Autodesk Fusion 360 part; units mm, degrees
(part 3 of 6)
  line L1098 (9.2939, 42.25) -> (5.0046, 42.25)
  line L1099 (4.1969, 48.5626) -> (3.4334, 47.8252)
  line L1100 (5.015, 40.75) -> (3.5, 40.75)
  line L1101 (3.5, 40.75) -> (2.5142, 47.7125)
  line L1102 (8.8126, 47.0763) -> (9.7083, 40.75)
  line L1103 (9.5063, 40.75) -> (9.2939, 42.25)
  line L1104 (8.5104, 47.0626) -> (9.274, 47.7999)
  line L1105 (10.1943, 47.9115) -> (9.4443, 47.9115)
  line L1106 (11.2083, 40.75) -> (10.2224, 47.7135)
  arc A162 (2.0758, 54.875) -> (1.5807, 54.3049) centre (2.0758, 54.375) ccw
  line L1107 (5.217, 40.75) -> (9.5063, 40.75)
  line L1108 (4.1602, 46.7869) -> (5.015, 40.75)
  line L1109 (9.4724, 47.7135) -> (8.8126, 47.0763)
  line L1110 (5.0046, 42.25) -> (5.217, 40.75)
  line L1111 (4.1717, 47.0626) -> (8.5104, 47.0626)
  line L1112 (9.4443, 47.9115) -> (8.5483, 48.8371)
  line L1113 (2.5142, 47.7125) -> (3.2642, 47.7125)
  line L1114 (10.2224, 47.7135) -> (9.4724, 47.7135)
  arc A163 (3.4391, 41.1799) -> (3.9342, 40.75) centre (3.9342, 41.25) ccw
  line L1115 (3.2358, 47.9125) -> (2.4858, 47.9125)
  line L1116 (7.4934, 54.875) -> (7.7058, 53.375)
  arc A164 (9.2692, 54.4451) -> (8.7741, 54.875) centre (8.7741, 54.375) ccw
  line L1117 (2.4858, 47.9125) -> (1.5, 54.875)
  line L1118 (3.4274, 53.375) -> (3.215, 54.875)
  line L1119 (9.2083, 54.875) -> (10.1943, 47.9115)
  line L1120 (3.4334, 47.8252) -> (4.1717, 47.0626)
  line L1121 (3.015, 54.875) -> (3.9088, 48.5624)
  line L1122 (9.274, 47.7999) -> (8.5357, 48.5626)
  line L1123 (8.5483, 48.8371) -> (7.6934, 54.875)
  line L1124 (3.215, 54.875) -> (7.4934, 54.875)
  line L1125 (8.5357, 48.5626) -> (4.1969, 48.5626)
  line L1126 (7.6934, 54.875) -> (9.2083, 54.875)
  line L1127 (3.9088, 48.5624) -> (3.2358, 47.9125)
  line L1128 (20.4138, 53.375) -> (16.1354, 53.375)
  line L1129 (15.723, 54.875) -> (14.208, 54.875)
  arc A165 (23.3405, 40.75) -> (23.8356, 41.3201) centre (23.3405, 41.25) ccw
  circle A166 centre (14.208, 41.625) radius 0.875
  line L1130 (15.9722, 47.7125) -> (16.8682, 46.7869)
  line L1131 (22.4163, 40.75) -> (23.9163, 40.75)
  line L1132 (22.0019, 42.25) -> (17.7126, 42.25)
  line L1133 (16.9049, 48.5626) -> (16.1414, 47.8252)
  line L1134 (17.723, 40.75) -> (16.208, 40.75)
  line L1135 (16.208, 40.75) -> (15.2222, 47.7125)
  line L1136 (21.5206, 47.0763) -> (22.4163, 40.75)
  line L1137 (22.2143, 40.75) -> (22.0019, 42.25)
  line L1138 (21.2184, 47.0626) -> (21.982, 47.7999)
  line L1139 (22.9023, 47.9115) -> (22.1523, 47.9115)
  line L1140 (23.9163, 40.75) -> (22.9304, 47.7135)
  arc A167 (14.7838, 54.875) -> (14.2887, 54.3049) centre (14.7838, 54.375) ccw
  line L1141 (17.925, 40.75) -> (22.2143, 40.75)
  line L1142 (16.8682, 46.7869) -> (17.723, 40.75)
  line L1143 (22.1804, 47.7135) -> (21.5206, 47.0763)
  line L1144 (17.7126, 42.25) -> (17.925, 40.75)
  line L1145 (16.8797, 47.0626) -> (21.2184, 47.0626)
  line L1146 (22.1523, 47.9115) -> (21.2563, 48.8371)
  line L1147 (15.2222, 47.7125) -> (15.9722, 47.7125)
  line L1148 (22.9304, 47.7135) -> (22.1804, 47.7135)
  arc A168 (16.1471, 41.1799) -> (16.6422, 40.75) centre (16.6422, 41.25) ccw
  line L1149 (15.9438, 47.9125) -> (15.1938, 47.9125)
  line L1150 (20.2014, 54.875) -> (20.4138, 53.375)
  arc A169 (21.9772, 54.4451) -> (21.4821, 54.875) centre (21.4821, 54.375) ccw
  line L1151 (15.1938, 47.9125) -> (14.208, 54.875)
  line L1152 (16.1354, 53.375) -> (15.923, 54.875)
  line L1153 (21.9163, 54.875) -> (22.9023, 47.9115)
  line L1154 (16.1414, 47.8252) -> (16.8797, 47.0626)
  line L1155 (15.723, 54.875) -> (16.6168, 48.5624)
  line L1156 (21.982, 47.7999) -> (21.2437, 48.5626)
  line L1157 (21.2563, 48.8371) -> (20.4014, 54.875)
  line L1158 (15.923, 54.875) -> (20.2014, 54.875)
  line L1159 (21.2437, 48.5626) -> (16.9049, 48.5626)
  line L1160 (20.4014, 54.875) -> (21.9163, 54.875)
  line L1161 (16.6168, 48.5624) -> (15.9438, 47.9125)
  line L1162 (33.1218, 53.375) -> (28.8434, 53.375)
  line L1163 (28.431, 54.875) -> (26.916, 54.875)
  arc A170 (36.0485, 40.75) -> (36.5436, 41.3201) centre (36.0485, 41.25) ccw
  circle A171 centre (26.916, 41.625) radius 0.875
  line L1164 (28.6802, 47.7125) -> (29.5762, 46.7869)
  line L1165 (35.1243, 40.75) -> (36.6243, 40.75)
  line L1166 (34.7099, 42.25) -> (30.4206, 42.25)
  line L1167 (29.6129, 48.5626) -> (28.8494, 47.8252)
  line L1168 (30.431, 40.75) -> (28.916, 40.75)
  line L1169 (28.916, 40.75) -> (27.9302, 47.7125)
  line L1170 (34.2286, 47.0763) -> (35.1243, 40.75)
  line L1171 (34.9223, 40.75) -> (34.7099, 42.25)
  line L1172 (33.9264, 47.0626) -> (34.69, 47.7999)
  line L1173 (35.6103, 47.9115) -> (34.8603, 47.9115)
  line L1174 (36.6243, 40.75) -> (35.6384, 47.7135)
  arc A172 (27.4918, 54.875) -> (26.9967, 54.3049) centre (27.4918, 54.375) ccw
  line L1175 (30.633, 40.75) -> (34.9223, 40.75)
  line L1176 (29.5762, 46.7869) -> (30.431, 40.75)
  line L1177 (34.8884, 47.7135) -> (34.2286, 47.0763)
  line L1178 (30.4206, 42.25) -> (30.633, 40.75)
  line L1179 (29.5877, 47.0626) -> (33.9264, 47.0626)
  line L1180 (34.8603, 47.9115) -> (33.9643, 48.8371)
  line L1181 (27.9302, 47.7125) -> (28.6802, 47.7125)
  line L1182 (35.6384, 47.7135) -> (34.8884, 47.7135)
  arc A173 (28.8551, 41.1799) -> (29.3502, 40.75) centre (29.3502, 41.25) ccw
  line L1183 (28.6518, 47.9125) -> (27.9018, 47.9125)
  line L1184 (32.9094, 54.875) -> (33.1218, 53.375)
  arc A174 (34.6852, 54.4451) -> (34.1901, 54.875) centre (34.1901, 54.375) ccw
  line L1185 (27.9018, 47.9125) -> (26.916, 54.875)
  line L1186 (28.8434, 53.375) -> (28.631, 54.875)
  line L1187 (34.6243, 54.875) -> (35.6103, 47.9115)
  line L1188 (28.8494, 47.8252) -> (29.5877, 47.0626)
  line L1189 (28.431, 54.875) -> (29.3248, 48.5624)
  line L1190 (34.69, 47.7999) -> (33.9517, 48.5626)
  line L1191 (33.9643, 48.8371) -> (33.1094, 54.875)
  line L1192 (28.631, 54.875) -> (32.9094, 54.875)
  line L1193 (33.9517, 48.5626) -> (29.6129, 48.5626)
  line L1194 (33.1094, 54.875) -> (34.6243, 54.875)
  line L1195 (29.3248, 48.5624) -> (28.6518, 47.9125)
  line L1196 (45.8298, 53.375) -> (41.5514, 53.375)
  line L1197 (41.139, 54.875) -> (39.624, 54.875)
  arc A175 (48.7565, 40.75) -> (49.2516, 41.3201) centre (48.7565, 41.25) ccw
  circle A176 centre (39.624, 41.625) radius 0.875
  line L1198 (41.3882, 47.7125) -> (42.2842, 46.7869)
  line L1199 (47.8323, 40.75) -> (49.3323, 40.75)
  line L1200 (47.4179, 42.25) -> (43.1286, 42.25)
  line L1201 (42.3209, 48.5626) -> (41.5574, 47.8252)
  line L1202 (43.139, 40.75) -> (41.624, 40.75)
  line L1203 (41.624, 40.75) -> (40.6382, 47.7125)
  line L1204 (46.9366, 47.0763) -> (47.8323, 40.75)
  line L1205 (47.6303, 40.75) -> (47.4179, 42.25)
  line L1206 (46.6344, 47.0626) -> (47.398, 47.7999)
  line L1207 (48.3183, 47.9115) -> (47.5683, 47.9115)
  line L1208 (49.3323, 40.75) -> (48.3464, 47.7135)
  arc A177 (40.1998, 54.875) -> (39.7047, 54.3049) centre (40.1998, 54.375) ccw
  line L1209 (43.341, 40.75) -> (47.6303, 40.75)
  line L1210 (42.2842, 46.7869) -> (43.139, 40.75)
  line L1211 (47.5964, 47.7135) -> (46.9366, 47.0763)
  line L1212 (43.1286, 42.25) -> (43.341, 40.75)
  line L1213 (42.2957, 47.0626) -> (46.6344, 47.0626)
  line L1214 (47.5683, 47.9115) -> (46.6723, 48.8371)
  line L1215 (40.6382, 47.7125) -> (41.3882, 47.7125)
  line L1216 (48.3464, 47.7135) -> (47.5964, 47.7135)
  arc A178 (41.5631, 41.1799) -> (42.0582, 40.75) centre (42.0582, 41.25) ccw
  line L1217 (41.3598, 47.9125) -> (40.6098, 47.9125)
  line L1218 (45.6174, 54.875) -> (45.8298, 53.375)
  arc A179 (47.3932, 54.4451) -> (46.8981, 54.875) centre (46.8981, 54.375) ccw
  line L1219 (40.6098, 47.9125) -> (39.624, 54.875)
  line L1220 (41.5514, 53.375) -> (41.339, 54.875)
  line L1221 (47.3323, 54.875) -> (48.3183, 47.9115)
  line L1222 (41.5574, 47.8252) -> (42.2957, 47.0626)
  line L1223 (41.139, 54.875) -> (42.0328, 48.5624)
  line L1224 (47.398, 47.7999) -> (46.6597, 48.5626)
  line L1225 (46.6723, 48.8371) -> (45.8174, 54.875)
  line L1226 (41.339, 54.875) -> (45.6174, 54.875)
  line L1227 (46.6597, 48.5626) -> (42.3209, 48.5626)
  line L1228 (45.8174, 54.875) -> (47.3323, 54.875)
  line L1229 (42.0328, 48.5624) -> (41.3598, 47.9125)
  line L1230 (58.5378, 53.375) -> (54.2594, 53.375)
  line L1231 (53.847, 54.875) -> (52.332, 54.875)
  arc A180 (61.4645, 40.75) -> (61.9596, 41.3201) centre (61.4645, 41.25) ccw
  circle A181 centre (52.332, 41.625) radius 0.875
  line L1232 (54.0962, 47.7125) -> (54.9922, 46.7869)
  line L1233 (60.5403, 40.75) -> (62.0403, 40.75)
  line L1234 (60.1259, 42.25) -> (55.8366, 42.25)
  line L1235 (55.0289, 48.5626) -> (54.2654, 47.8252)
  line L1236 (55.847, 40.75) -> (54.332, 40.75)
  line L1237 (54.332, 40.75) -> (53.3462, 47.7125)
  line L1238 (59.6446, 47.0763) -> (60.5403, 40.75)
  line L1239 (60.3383, 40.75) -> (60.1259, 42.25)
  line L1240 (59.3424, 47.0626) -> (60.106, 47.7999)
  line L1241 (61.0263, 47.9115) -> (60.2763, 47.9115)
  line L1242 (62.0403, 40.75) -> (61.0544, 47.7135)
  arc A182 (52.9078, 54.875) -> (52.4127, 54.3049) centre (52.9078, 54.375) ccw
  line L1243 (56.049, 40.75) -> (60.3383, 40.75)
  line L1244 (54.9922, 46.7869) -> (55.847, 40.75)
  line L1245 (60.3044, 47.7135) -> (59.6446, 47.0763)
  line L1246 (55.8366, 42.25) -> (56.049, 40.75)
  line L1247 (55.0037, 47.0626) -> (59.3424, 47.0626)
  line L1248 (60.2763, 47.9115) -> (59.3803, 48.8371)
  line L1249 (53.3462, 47.7125) -> (54.0962, 47.7125)
  line L1250 (61.0544, 47.7135) -> (60.3044, 47.7135)
  arc A183 (54.2711, 41.1799) -> (54.7662, 40.75) centre (54.7662, 41.25) ccw
  line L1251 (54.0678, 47.9125) -> (53.3178, 47.9125)
  line L1252 (58.3254, 54.875) -> (58.5378, 53.375)
  arc A184 (60.1012, 54.4451) -> (59.6061, 54.875) centre (59.6061, 54.375) ccw
  line L1253 (53.3178, 47.9125) -> (52.332, 54.875)
  line L1254 (54.2594, 53.375) -> (54.047, 54.875)
  line L1255 (60.0403, 54.875) -> (61.0263, 47.9115)
  line L1256 (54.2654, 47.8252) -> (55.0037, 47.0626)
  line L1257 (53.847, 54.875) -> (54.7408, 48.5624)
  line L1258 (60.106, 47.7999) -> (59.3677, 48.5626)
  line L1259 (59.3803, 48.8371) -> (58.5254, 54.875)
  line L1260 (54.047, 54.875) -> (58.3254, 54.875)
  line L1261 (59.3677, 48.5626) -> (55.0289, 48.5626)
  line L1262 (58.5254, 54.875) -> (60.0403, 54.875)
  line L1263 (54.7408, 48.5624) -> (54.0678, 47.9125)
  line L1264 (71.2458, 53.375) -> (66.9674, 53.375)
  line L1265 (66.555, 54.875) -> (65.04, 54.875)
  arc A185 (74.1725, 40.75) -> (74.6676, 41.3201) centre (74.1725, 41.25) ccw
  circle A186 centre (65.04, 41.625) radius 0.875
  line L1266 (66.8042, 47.7125) -> (67.7002, 46.7869)
  line L1267 (73.2483, 40.75) -> (74.7483, 40.75)
  line L1268 (72.8339, 42.25) -> (68.5446, 42.25)
  line L1269 (67.7369, 48.5626) -> (66.9734, 47.8252)
  line L1270 (68.555, 40.75) -> (67.04, 40.75)
  line L1271 (67.04, 40.75) -> (66.0542, 47.7125)
  line L1272 (72.3526, 47.0763) -> (73.2483, 40.75)
  line L1273 (73.0463, 40.75) -> (72.8339, 42.25)
  line L1274 (72.0504, 47.0626) -> (72.814, 47.7999)
  line L1275 (73.7343, 47.9115) -> (72.9843, 47.9115)
  line L1276 (74.7483, 40.75) -> (73.7624, 47.7135)
  arc A187 (65.6158, 54.875) -> (65.1207, 54.3049) centre (65.6158, 54.375) ccw
  line L1277 (68.757, 40.75) -> (73.0463, 40.75)
  line L1278 (67.7002, 46.7869) -> (68.555, 40.75)
  line L1279 (73.0124, 47.7135) -> (72.3526, 47.0763)
  line L1280 (68.5446, 42.25) -> (68.757, 40.75)
  line L1281 (67.7117, 47.0626) -> (72.0504, 47.0626)
  line L1282 (72.9843, 47.9115) -> (72.0883, 48.8371)
  line L1283 (66.0542, 47.7125) -> (66.8042, 47.7125)
  line L1284 (73.7624, 47.7135) -> (73.0124, 47.7135)
  arc A188 (66.9791, 41.1799) -> (67.4742, 40.75) centre (67.4742, 41.25) ccw
  line L1285 (66.7758, 47.9125) -> (66.0258, 47.9125)
  line L1286 (71.0334, 54.875) -> (71.2458, 53.375)
  arc A189 (72.8092, 54.4451) -> (72.3141, 54.875) centre (72.3141, 54.375) ccw
  line L1287 (66.0258, 47.9125) -> (65.04, 54.875)
  line L1288 (66.9674, 53.375) -> (66.755, 54.875)
  line L1289 (72.7483, 54.875) -> (73.7343, 47.9115)
  line L1290 (66.9734, 47.8252) -> (67.7117, 47.0626)
  line L1291 (66.555, 54.875) -> (67.4488, 48.5624)
  line L1292 (72.814, 47.7999) -> (72.0757, 48.5626)
  line L1293 (72.0883, 48.8371) -> (71.2334, 54.875)
  line L1294 (66.755, 54.875) -> (71.0334, 54.875)
  line L1295 (72.0757, 48.5626) -> (67.7369, 48.5626)
  line L1296 (71.2334, 54.875) -> (72.7483, 54.875)
  line L1297 (67.4488, 48.5624) -> (66.7758, 47.9125)
  line L1298 (83.9538, 53.375) -> (79.6754, 53.375)
  line L1299 (79.263, 54.875) -> (77.748, 54.875)
  arc A190 (86.8805, 40.75) -> (87.3756, 41.3201) centre (86.8805, 41.25) ccw
  circle A191 centre (77.748, 41.625) radius 0.875
  line L1300 (79.5122, 47.7125) -> (80.4082, 46.7869)
  line L1301 (85.9563, 40.75) -> (87.4563, 40.75)
  line L1302 (85.5419, 42.25) -> (81.2526, 42.25)
  line L1303 (80.4449, 48.5626) -> (79.6814, 47.8252)
  line L1304 (81.263, 40.75) -> (79.748, 40.75)
  line L1305 (79.748, 40.75) -> (78.7622, 47.7125)
  line L1306 (85.0606, 47.0763) -> (85.9563, 40.75)
  line L1307 (85.7543, 40.75) -> (85.5419, 42.25)
  line L1308 (84.7584, 47.0626) -> (85.522, 47.7999)
  line L1309 (86.4423, 47.9115) -> (85.6923, 47.9115)
  line L1310 (87.4563, 40.75) -> (86.4704, 47.7135)
  arc A192 (78.3238, 54.875) -> (77.8287, 54.3049) centre (78.3238, 54.375) ccw
  line L1311 (81.465, 40.75) -> (85.7543, 40.75)
  line L1312 (80.4082, 46.7869) -> (81.263, 40.75)
  line L1313 (85.7204, 47.7135) -> (85.0606, 47.0763)
  line L1314 (81.2526, 42.25) -> (81.465, 40.75)
  line L1315 (80.4197, 47.0626) -> (84.7584, 47.0626)
  line L1316 (85.6923, 47.9115) -> (84.7963, 48.8371)
  line L1317 (78.7622, 47.7125) -> (79.5122, 47.7125)
  line L1318 (86.4704, 47.7135) -> (85.7204, 47.7135)
  arc A193 (79.6871, 41.1799) -> (80.1822, 40.75) centre (80.1822, 41.25) ccw
  line L1319 (79.4838, 47.9125) -> (78.7338, 47.9125)
  line L1320 (83.7414, 54.875) -> (83.9538, 53.375)
  arc A194 (85.5172, 54.4451) -> (85.0221, 54.875) centre (85.0221, 54.375) ccw
  line L1321 (78.7338, 47.9125) -> (77.748, 54.875)
  line L1322 (79.6754, 53.375) -> (79.463, 54.875)
  line L1323 (85.4563, 54.875) -> (86.4423, 47.9115)
  line L1324 (79.6814, 47.8252) -> (80.4197, 47.0626)
  line L1325 (79.263, 54.875) -> (80.1568, 48.5624)
  line L1326 (85.522, 47.7999) -> (84.7837, 48.5626)
  line L1327 (84.7963, 48.8371) -> (83.9414, 54.875)
  line L1328 (79.463, 54.875) -> (83.7414, 54.875)
  line L1329 (84.7837, 48.5626) -> (80.4449, 48.5626)
  line L1330 (83.9414, 54.875) -> (85.4563, 54.875)
  line L1331 (80.1568, 48.5624) -> (79.4838, 47.9125)
  line L1332 (96.6618, 53.375) -> (92.3834, 53.375)
  line L1333 (91.971, 54.875) -> (90.456, 54.875)
  arc A195 (99.5885, 40.75) -> (100.0836, 41.3201) centre (99.5885, 41.25) ccw
  circle A196 centre (90.456, 41.625) radius 0.875
  line L1334 (92.2202, 47.7125) -> (93.1162, 46.7869)
  line L1335 (98.6643, 40.75) -> (100.1643, 40.75)
  line L1336 (98.2499, 42.25) -> (93.9606, 42.25)
  line L1337 (93.1529, 48.5626) -> (92.3894, 47.8252)
  line L1338 (93.971, 40.75) -> (92.456, 40.75)
  line L1339 (92.456, 40.75) -> (91.4702, 47.7125)
  line L1340 (97.7686, 47.0763) -> (98.6643, 40.75)
  line L1341 (98.4623, 40.75) -> (98.2499, 42.25)
  line L1342 (97.4664, 47.0626) -> (98.23, 47.7999)
  line L1343 (99.1503, 47.9115) -> (98.4003, 47.9115)
  line L1344 (100.1643, 40.75) -> (99.1784, 47.7135)
  arc A197 (91.0318, 54.875) -> (90.5367, 54.3049) centre (91.0318, 54.375) ccw
  line L1345 (94.173, 40.75) -> (98.4623, 40.75)
  line L1346 (93.1162, 46.7869) -> (93.971, 40.75)
  line L1347 (98.4284, 47.7135) -> (97.7686, 47.0763)
  line L1348 (93.9606, 42.25) -> (94.173, 40.75)
  line L1349 (93.1277, 47.0626) -> (97.4664, 47.0626)
  line L1350 (98.4003, 47.9115) -> (97.5043, 48.8371)
  line L1351 (91.4702, 47.7125) -> (92.2202, 47.7125)
  line L1352 (99.1784, 47.7135) -> (98.4284, 47.7135)
  arc A198 (92.3951, 41.1799) -> (92.8902, 40.75) centre (92.8902, 41.25) ccw
  line L1353 (92.1918, 47.9125) -> (91.4418, 47.9125)
  line L1354 (96.4494, 54.875) -> (96.6618, 53.375)
  arc A199 (98.2252, 54.4451) -> (97.7301, 54.875) centre (97.7301, 54.375) ccw
  line L1355 (91.4418, 47.9125) -> (90.456, 54.875)
  line L1356 (92.3834, 53.375) -> (92.171, 54.875)
  line L1357 (98.1643, 54.875) -> (99.1503, 47.9115)
  line L1358 (92.3894, 47.8252) -> (93.1277, 47.0626)
  line L1359 (91.971, 54.875) -> (92.8648, 48.5624)
  line L1360 (98.23, 47.7999) -> (97.4917, 48.5626)
  line L1361 (97.5043, 48.8371) -> (96.6494, 54.875)
  line L1362 (92.171, 54.875) -> (96.4494, 54.875)
  line L1363 (97.4917, 48.5626) -> (93.1529, 48.5626)
  line L1364 (96.6494, 54.875) -> (98.1643, 54.875)
  line L1365 (92.8648, 48.5624) -> (92.1918, 47.9125)
  line L1366 (109.3698, 53.375) -> (105.0914, 53.375)
  line L1367 (104.679, 54.875) -> (103.164, 54.875)
  arc A200 (112.2965, 40.75) -> (112.7916, 41.3201) centre (112.2965, 41.25) ccw
  circle A201 centre (103.164, 41.625) radius 0.875
  line L1368 (104.9282, 47.7125) -> (105.8242, 46.7869)
  line L1369 (111.3723, 40.75) -> (112.8723, 40.75)
  line L1370 (110.9579, 42.25) -> (106.6686, 42.25)
  line L1371 (105.8609, 48.5626) -> (105.0974, 47.8252)
  line L1372 (106.679, 40.75) -> (105.164, 40.75)
  line L1373 (105.164, 40.75) -> (104.1782, 47.7125)
  line L1374 (110.4766, 47.0763) -> (111.3723, 40.75)
  line L1375 (111.1703, 40.75) -> (110.9579, 42.25)
  line L1376 (110.1744, 47.0626) -> (110.938, 47.7999)
  line L1377 (111.8583, 47.9115) -> (111.1083, 47.9115)
  line L1378 (112.8723, 40.75) -> (111.8864, 47.7135)
  arc A202 (103.7398, 54.875) -> (103.2447, 54.3049) centre (103.7398, 54.375) ccw
  line L1379 (106.881, 40.75) -> (111.1703, 40.75)
  line L1380 (105.8242, 46.7869) -> (106.679, 40.75)
  line L1381 (111.1364, 47.7135) -> (110.4766, 47.0763)
  line L1382 (106.6686, 42.25) -> (106.881, 40.75)
  line L1383 (105.8357, 47.0626) -> (110.1744, 47.0626)
  line L1384 (111.1083, 47.9115) -> (110.2123, 48.8371)
  line L1385 (104.1782, 47.7125) -> (104.9282, 47.7125)
  line L1386 (111.8864, 47.7135) -> (111.1364, 47.7135)
  arc A203 (105.1031, 41.1799) -> (105.5982, 40.75) centre (105.5982, 41.25) ccw
  line L1387 (104.8998, 47.9125) -> (104.1498, 47.9125)
  line L1388 (109.1574, 54.875) -> (109.3698, 53.375)
  arc A204 (110.9332, 54.4451) -> (110.4381, 54.875) centre (110.4381, 54.375) ccw
  line L1389 (104.1498, 47.9125) -> (103.164, 54.875)
  line L1390 (105.0914, 53.375) -> (104.879, 54.875)
  line L1391 (110.8723, 54.875) -> (111.8583, 47.9115)
  line L1392 (105.0974, 47.8252) -> (105.8357, 47.0626)
  line L1393 (104.679, 54.875) -> (105.5728, 48.5624)
  line L1394 (110.938, 47.7999) -> (110.1997, 48.5626)
  line L1395 (110.2123, 48.8371) -> (109.3574, 54.875)
  line L1396 (104.879, 54.875) -> (109.1574, 54.875)
  line L1397 (110.1997, 48.5626) -> (105.8609, 48.5626)
  line L1398 (109.3574, 54.875) -> (110.8723, 54.875)
  line L1399 (105.5728, 48.5624) -> (104.8998, 47.9125)
  line L1400 (122.0778, 53.375) -> (117.7994, 53.375)
  line L1401 (117.387, 54.875) -> (115.872, 54.875)
  arc A205 (125.0045, 40.75) -> (125.4996, 41.3201) centre (125.0045, 41.25) ccw
  circle A206 centre (115.872, 41.625) radius 0.875
  line L1402 (117.6362, 47.7125) -> (118.5322, 46.7869)
  line L1403 (124.0803, 40.75) -> (125.5803, 40.75)
  line L1404 (123.6659, 42.25) -> (119.3766, 42.25)
  line L1405 (118.5689, 48.5626) -> (117.8054, 47.8252)
  line L1406 (119.387, 40.75) -> (117.872, 40.75)
  line L1407 (117.872, 40.75) -> (116.8862, 47.7125)
  line L1408 (123.1846, 47.0763) -> (124.0803, 40.75)
  line L1409 (123.8783, 40.75) -> (123.6659, 42.25)
  line L1410 (122.8824, 47.0626) -> (123.646, 47.7999)
  line L1411 (124.5663, 47.9115) -> (123.8163, 47.9115)
  line L1412 (125.5803, 40.75) -> (124.5944, 47.7135)
  arc A207 (116.4478, 54.875) -> (115.9527, 54.3049) centre (116.4478, 54.375) ccw
  line L1413 (119.589, 40.75) -> (123.8783, 40.75)
  line L1414 (118.5322, 46.7869) -> (119.387, 40.75)
  line L1415 (123.8444, 47.7135) -> (123.1846, 47.0763)
  line L1416 (119.3766, 42.25) -> (119.589, 40.75)
  line L1417 (118.5437, 47.0626) -> (122.8824, 47.0626)
  line L1418 (123.8163, 47.9115) -> (122.9203, 48.8371)
  line L1419 (116.8862, 47.7125) -> (117.6362, 47.7125)
  line L1420 (124.5944, 47.7135) -> (123.8444, 47.7135)
  arc A208 (117.8111, 41.1799) -> (118.3062, 40.75) centre (118.3062, 41.25) ccw
  line L1421 (117.6078, 47.9125) -> (116.8578, 47.9125)
  line L1422 (121.8654, 54.875) -> (122.0778, 53.375)
  arc A209 (123.6412, 54.4451) -> (123.1461, 54.875) centre (123.1461, 54.375) ccw
  line L1423 (116.8578, 47.9125) -> (115.872, 54.875)
  line L1424 (117.7994, 53.375) -> (117.587, 54.875)
  line L1425 (123.5803, 54.875) -> (124.5663, 47.9115)
  line L1426 (117.8054, 47.8252) -> (118.5437, 47.0626)
  line L1427 (117.387, 54.875) -> (118.2808, 48.5624)
  line L1428 (123.646, 47.7999) -> (122.9077, 48.5626)
  line L1429 (122.9203, 48.8371) -> (122.0654, 54.875)
  line L1430 (117.587, 54.875) -> (121.8654, 54.875)
  line L1431 (122.9077, 48.5626) -> (118.5689, 48.5626)
  line L1432 (122.0654, 54.875) -> (123.5803, 54.875)
  line L1433 (118.2808, 48.5624) -> (117.6078, 47.9125)
  line L1434 (134.7858, 53.375) -> (130.5074, 53.375)
  line L1435 (130.095, 54.875) -> (128.58, 54.875)
  arc A210 (137.7125, 40.75) -> (138.2076, 41.3201) centre (137.7125, 41.25) ccw
  circle A211 centre (128.58, 41.625) radius 0.875
  line L1436 (130.3442, 47.7125) -> (131.2402, 46.7869)
  line L1437 (136.7883, 40.75) -> (138.2883, 40.75)
  line L1438 (136.3739, 42.25) -> (132.0846, 42.25)
  line L1439 (131.2769, 48.5626) -> (130.5134, 47.8252)
  line L1440 (132.095, 40.75) -> (130.58, 40.75)
  line L1441 (130.58, 40.75) -> (129.5942, 47.7125)
  line L1442 (135.8926, 47.0763) -> (136.7883, 40.75)
  line L1443 (136.5863, 40.75) -> (136.3739, 42.25)
  line L1444 (135.5904, 47.0626) -> (136.354, 47.7999)
  line L1445 (137.2743, 47.9115) -> (136.5243, 47.9115)
  line L1446 (138.2883, 40.75) -> (137.3024, 47.7135)
  arc A212 (129.1558, 54.875) -> (128.6607, 54.3049) centre (129.1558, 54.375) ccw
  line L1447 (132.297, 40.75) -> (136.5863, 40.75)
  line L1448 (131.2402, 46.7869) -> (132.095, 40.75)
  line L1449 (136.5524, 47.7135) -> (135.8926, 47.0763)
  line L1450 (132.0846, 42.25) -> (132.297, 40.75)
  line L1451 (131.2517, 47.0626) -> (135.5904, 47.0626)
  line L1452 (136.5243, 47.9115) -> (135.6283, 48.8371)
  line L1453 (129.5942, 47.7125) -> (130.3442, 47.7125)
  line L1454 (137.3024, 47.7135) -> (136.5524, 47.7135)
  arc A213 (130.5191, 41.1799) -> (131.0142, 40.75) centre (131.0142, 41.25) ccw
  line L1455 (130.3158, 47.9125) -> (129.5658, 47.9125)
  line L1456 (134.5734, 54.875) -> (134.7858, 53.375)
  arc A214 (136.3492, 54.4451) -> (135.8541, 54.875) centre (135.8541, 54.375) ccw
  line L1457 (129.5658, 47.9125) -> (128.58, 54.875)
  line L1458 (130.5074, 53.375) -> (130.295, 54.875)
  line L1459 (136.2883, 54.875) -> (137.2743, 47.9115)
  line L1460 (130.5134, 47.8252) -> (131.2517, 47.0626)
  line L1461 (130.095, 54.875) -> (130.9888, 48.5624)
  line L1462 (136.354, 47.7999) -> (135.6157, 48.5626)
  line L1463 (135.6283, 48.8371) -> (134.7734, 54.875)
  line L1464 (130.295, 54.875) -> (134.5734, 54.875)
  line L1465 (135.6157, 48.5626) -> (131.2769, 48.5626)
  line L1466 (134.7734, 54.875) -> (136.2883, 54.875)
  line L1467 (130.9888, 48.5624) -> (130.3158, 47.9125)
  line L1468 (147.4938, 53.375) -> (143.2154, 53.375)
  line L1469 (142.803, 54.875) -> (141.288, 54.875)
  arc A215 (150.4205, 40.75) -> (150.9156, 41.3201) centre (150.4205, 41.25) ccw
  circle A216 centre (141.288, 41.625) radius 0.875
  line L1470 (143.0522, 47.7125) -> (143.9482, 46.7869)
  line L1471 (149.4963, 40.75) -> (150.9963, 40.75)
  line L1472 (149.0819, 42.25) -> (144.7926, 42.25)
  line L1473 (143.9849, 48.5626) -> (143.2214, 47.8252)
  line L1474 (144.803, 40.75) -> (143.288, 40.75)
  line L1475 (143.288, 40.75) -> (142.3022, 47.7125)
  line L1476 (148.6006, 47.0763) -> (149.4963, 40.75)
  line L1477 (149.2943, 40.75) -> (149.0819, 42.25)
  line L1478 (148.2984, 47.0626) -> (149.062, 47.7999)
  line L1479 (149.9823, 47.9115) -> (149.2323, 47.9115)
  line L1480 (150.9963, 40.75) -> (150.0104, 47.7135)
  arc A217 (141.8638, 54.875) -> (141.3687, 54.3049) centre (141.8638, 54.375) ccw
  line L1481 (145.005, 40.75) -> (149.2943, 40.75)
  line L1482 (143.9482, 46.7869) -> (144.803, 40.75)
  line L1483 (149.2604, 47.7135) -> (148.6006, 47.0763)
  line L1484 (144.7926, 42.25) -> (145.005, 40.75)
  line L1485 (143.9597, 47.0626) -> (148.2984, 47.0626)
  line L1486 (149.2323, 47.9115) -> (148.3363, 48.8371)
  line L1487 (142.3022, 47.7125) -> (143.0522, 47.7125)
  line L1488 (150.0104, 47.7135) -> (149.2604, 47.7135)
  arc A218 (143.2271, 41.1799) -> (143.7222, 40.75) centre (143.7222, 41.25) ccw
  line L1489 (143.0238, 47.9125) -> (142.2738, 47.9125)
  line L1490 (147.2814, 54.875) -> (147.4938, 53.375)
  arc A219 (149.0572, 54.4451) -> (148.5621, 54.875) centre (148.5621, 54.375) ccw
  line L1491 (142.2738, 47.9125) -> (141.288, 54.875)
  line L1492 (143.2154, 53.375) -> (143.003, 54.875)
  line L1493 (148.9963, 54.875) -> (149.9823, 47.9115)
  line L1494 (143.2214, 47.8252) -> (143.9597, 47.0626)
  line L1495 (142.803, 54.875) -> (143.6968, 48.5624)
  line L1496 (149.062, 47.7999) -> (148.3237, 48.5626)
  line L1497 (148.3363, 48.8371) -> (147.4814, 54.875)
  line L1498 (143.003, 54.875) -> (147.2814, 54.875)
  line L1499 (148.3237, 48.5626) -> (143.9849, 48.5626)
  line L1500 (147.4814, 54.875) -> (148.9963, 54.875)
  line L1501 (143.6968, 48.5624) -> (143.0238, 47.9125)
  line L1502 (160.2018, 53.375) -> (155.9234, 53.375)
  line L1503 (155.511, 54.875) -> (153.996, 54.875)
  arc A220 (163.1285, 40.75) -> (163.6236, 41.3201) centre (163.1285, 41.25) ccw
  circle A221 centre (153.996, 41.625) radius 0.875
  line L1504 (155.7602, 47.7125) -> (156.6562, 46.7869)
  line L1505 (162.2043, 40.75) -> (163.7043, 40.75)
  line L1506 (161.7899, 42.25) -> (157.5006, 42.25)
  line L1507 (156.6929, 48.5626) -> (155.9294, 47.8252)
  line L1508 (157.511, 40.75) -> (155.996, 40.75)
  line L1509 (155.996, 40.75) -> (155.0102, 47.7125)
  line L1510 (161.3086, 47.0763) -> (162.2043, 40.75)
  line L1511 (162.0023, 40.75) -> (161.7899, 42.25)
  line L1512 (161.0064, 47.0626) -> (161.77, 47.7999)
  line L1513 (162.6903, 47.9115) -> (161.9403, 47.9115)
  line L1514 (163.7043, 40.75) -> (162.7184, 47.7135)
  arc A222 (154.5718, 54.875) -> (154.0767, 54.3049) centre (154.5718, 54.375) ccw
  line L1515 (157.713, 40.75) -> (162.0023, 40.75)
  line L1516 (156.6562, 46.7869) -> (157.511, 40.75)
  line L1517 (161.9684, 47.7135) -> (161.3086, 47.0763)
  line L1518 (157.5006, 42.25) -> (157.713, 40.75)
  line L1519 (156.6677, 47.0626) -> (161.0064, 47.0626)
  line L1520 (161.9403, 47.9115) -> (161.0443, 48.8371)
  line L1521 (155.0102, 47.7125) -> (155.7602, 47.7125)
  line L1522 (162.7184, 47.7135) -> (161.9684, 47.7135)
  arc A223 (155.9351, 41.1799) -> (156.4302, 40.75) centre (156.4302, 41.25) ccw
  line L1523 (155.7318, 47.9125) -> (154.9818, 47.9125)
  line L1524 (159.9894, 54.875) -> (160.2018, 53.375)
  arc A224 (161.7652, 54.4451) -> (161.2701, 54.875) centre (161.2701, 54.375) ccw
  line L1525 (154.9818, 47.9125) -> (153.996, 54.875)
  line L1526 (155.9234, 53.375) -> (155.711, 54.875)
  line L1527 (161.7043, 54.875) -> (162.6903, 47.9115)
  line L1528 (155.9294, 47.8252) -> (156.6677, 47.0626)
  line L1529 (155.511, 54.875) -> (156.4048, 48.5624)
  line L1530 (161.77, 47.7999) -> (161.0317, 48.5626)
  line L1531 (161.0443, 48.8371) -> (160.1894, 54.875)
  line L1532 (155.711, 54.875) -> (159.9894, 54.875)
  line L1533 (161.0317, 48.5626) -> (156.6929, 48.5626)
  line L1534 (160.1894, 54.875) -> (161.7043, 54.875)
  line L1535 (156.4048, 48.5624) -> (155.7318, 47.9125)
  line L1536 (172.9098, 53.375) -> (168.6314, 53.375)
  line L1537 (168.219, 54.875) -> (166.704, 54.875)
  arc A225 (175.8365, 40.75) -> (176.3316, 41.3201) centre (175.8365, 41.25) ccw
  circle A226 centre (166.704, 41.625) radius 0.875
  line L1538 (168.4682, 47.7125) -> (169.3642, 46.7869)
  line L1539 (174.9123, 40.75) -> (176.4123, 40.75)
  line L1540 (174.4979, 42.25) -> (170.2086, 42.25)
  line L1541 (169.4009, 48.5626) -> (168.6374, 47.8252)
  line L1542 (170.219, 40.75) -> (168.704, 40.75)
  line L1543 (168.704, 40.75) -> (167.7182, 47.7125)
  line L1544 (174.0166, 47.0763) -> (174.9123, 40.75)
  line L1545 (174.7103, 40.75) -> (174.4979, 42.25)
  line L1546 (173.7144, 47.0626) -> (174.478, 47.7999)
  line L1547 (175.3983, 47.9115) -> (174.6483, 47.9115)
  line L1548 (176.4123, 40.75) -> (175.4264, 47.7135)
  arc A227 (167.2798, 54.875) -> (166.7847, 54.3049) centre (167.2798, 54.375) ccw
  line L1549 (170.421, 40.75) -> (174.7103, 40.75)
  line L1550 (169.3642, 46.7869) -> (170.219, 40.75)
  line L1551 (174.6764, 47.7135) -> (174.0166, 47.0763)
  line L1552 (170.2086, 42.25) -> (170.421, 40.75)
  line L1553 (169.3757, 47.0626) -> (173.7144, 47.0626)
  line L1554 (174.6483, 47.9115) -> (173.7523, 48.8371)
  line L1555 (167.7182, 47.7125) -> (168.4682, 47.7125)
  line L1556 (175.4264, 47.7135) -> (174.6764, 47.7135)
  arc A228 (168.6431, 41.1799) -> (169.1382, 40.75) centre (169.1382, 41.25) ccw
  line L1557 (168.4398, 47.9125) -> (167.6898, 47.9125)
  line L1558 (172.6974, 54.875) -> (172.9098, 53.375)
  arc A229 (174.4732, 54.4451) -> (173.9781, 54.875) centre (173.9781, 54.375) ccw
  line L1559 (167.6898, 47.9125) -> (166.704, 54.875)
  line L1560 (168.6314, 53.375) -> (168.419, 54.875)
  line L1561 (174.4123, 54.875) -> (175.3983, 47.9115)
  line L1562 (168.6374, 47.8252) -> (169.3757, 47.0626)
  line L1563 (168.219, 54.875) -> (169.1128, 48.5624)
  line L1564 (174.478, 47.7999) -> (173.7397, 48.5626)
  line L1565 (173.7523, 48.8371) -> (172.8974, 54.875)
  line L1566 (168.419, 54.875) -> (172.6974, 54.875)
  line L1567 (173.7397, 48.5626) -> (169.4009, 48.5626)
  line L1568 (172.8974, 54.875) -> (174.4123, 54.875)
  line L1569 (169.1128, 48.5624) -> (168.4398, 47.9125)
  line L1570 (185.6178, 53.375) -> (181.3394, 53.375)
  line L1571 (180.927, 54.875) -> (179.412, 54.875)
  arc A230 (188.5445, 40.75) -> (189.0396, 41.3201) centre (188.5445, 41.25) ccw
  circle A231 centre (179.412, 41.625) radius 0.875
  line L1572 (181.1762, 47.7125) -> (182.0722, 46.7869)
  line L1573 (187.6203, 40.75) -> (189.1203, 40.75)
  line L1574 (187.2059, 42.25) -> (182.9166, 42.25)
  line L1575 (182.1089, 48.5626) -> (181.3454, 47.8252)
  line L1576 (182.927, 40.75) -> (181.412, 40.75)
  line L1577 (181.412, 40.75) -> (180.4262, 47.7125)
  line L1578 (186.7246, 47.0763) -> (187.6203, 40.75)
  line L1579 (187.4183, 40.75) -> (187.2059, 42.25)
  line L1580 (186.4224, 47.0626) -> (187.186, 47.7999)
  line L1581 (188.1063, 47.9115) -> (187.3563, 47.9115)
  line L1582 (189.1203, 40.75) -> (188.1344, 47.7135)
  arc A232 (179.9878, 54.875) -> (179.4927, 54.3049) centre (179.9878, 54.375) ccw
  line L1583 (183.129, 40.75) -> (187.4183, 40.75)
  line L1584 (182.0722, 46.7869) -> (182.927, 40.75)
  line L1585 (187.3844, 47.7135) -> (186.7246, 47.0763)
  line L1586 (182.9166, 42.25) -> (183.129, 40.75)
  line L1587 (182.0837, 47.0626) -> (186.4224, 47.0626)
  line L1588 (187.3563, 47.9115) -> (186.4603, 48.8371)
  line L1589 (180.4262, 47.7125) -> (181.1762, 47.7125)
  line L1590 (188.1344, 47.7135) -> (187.3844, 47.7135)
  arc A233 (181.3511, 41.1799) -> (181.8462, 40.75) centre (181.8462, 41.25) ccw
  line L1591 (181.1478, 47.9125) -> (180.3978, 47.9125)
  line L1592 (185.4054, 54.875) -> (185.6178, 53.375)
  arc A234 (187.1812, 54.4451) -> (186.6861, 54.875) centre (186.6861, 54.375) ccw
  line L1593 (180.3978, 47.9125) -> (179.412, 54.875)
  line L1594 (181.3394, 53.375) -> (181.127, 54.875)
  line L1595 (187.1203, 54.875) -> (188.1063, 47.9115)
  line L1596 (181.3454, 47.8252) -> (182.0837, 47.0626)
  line L1597 (180.927, 54.875) -> (181.8208, 48.5624)
  line L1598 (187.186, 47.7999) -> (186.4477, 48.5626)
  line L1599 (186.4603, 48.8371) -> (185.6054, 54.875)
  line L1600 (181.127, 54.875) -> (185.4054, 54.875)
  line L1601 (186.4477, 48.5626) -> (182.1089, 48.5626)
  line L1602 (185.6054, 54.875) -> (187.1203, 54.875)
  line L1603 (181.8208, 48.5624) -> (181.1478, 47.9125)
  line L1604 (198.3258, 53.375) -> (194.0474, 53.375)
  line L1605 (193.635, 54.875) -> (192.12, 54.875)
  arc A235 (201.2525, 40.75) -> (201.7476, 41.3201) centre (201.2525, 41.25) ccw
  circle A236 centre (192.12, 41.625) radius 0.875
  line L1606 (193.8842, 47.7125) -> (194.7802, 46.7869)
  line L1607 (200.3283, 40.75) -> (201.8283, 40.75)
  line L1608 (199.9139, 42.25) -> (195.6246, 42.25)
  line L1609 (194.8169, 48.5626) -> (194.0534, 47.8252)
  line L1610 (195.635, 40.75) -> (194.12, 40.75)
  line L1611 (194.12, 40.75) -> (193.1342, 47.7125)
  line L1612 (199.4326, 47.0763) -> (200.3283, 40.75)
  line L1613 (200.1263, 40.75) -> (199.9139, 42.25)
  line L1614 (199.1304, 47.0626) -> (199.894, 47.7999)
  line L1615 (200.8143, 47.9115) -> (200.0643, 47.9115)
  line L1616 (201.8283, 40.75) -> (200.8424, 47.7135)
  arc A237 (192.6958, 54.875) -> (192.2007, 54.3049) centre (192.6958, 54.375) ccw
  line L1617 (195.837, 40.75) -> (200.1263, 40.75)
  line L1618 (194.7802, 46.7869) -> (195.635, 40.75)
  line L1619 (200.0924, 47.7135) -> (199.4326, 47.0763)
  line L1620 (195.6246, 42.25) -> (195.837, 40.75)
  line L1621 (194.7917, 47.0626) -> (199.1304, 47.0626)
  line L1622 (200.0643, 47.9115) -> (199.1683, 48.8371)
  line L1623 (193.1342, 47.7125) -> (193.8842, 47.7125)
  line L1624 (200.8424, 47.7135) -> (200.0924, 47.7135)
  arc A238 (194.0591, 41.1799) -> (194.5542, 40.75) centre (194.5542, 41.25) ccw
  line L1625 (193.8558, 47.9125) -> (193.1058, 47.9125)
  line L1626 (198.1134, 54.875) -> (198.3258, 53.375)
  arc A239 (199.8892, 54.4451) -> (199.3941, 54.875) centre (199.3941, 54.375) ccw
  line L1627 (193.1058, 47.9125) -> (192.12, 54.875)
  line L1628 (194.0474, 53.375) -> (193.835, 54.875)
  line L1629 (199.8283, 54.875) -> (200.8143, 47.9115)
  line L1630 (194.0534, 47.8252) -> (194.7917, 47.0626)
  line L1631 (193.635, 54.875) -> (194.5288, 48.5624)
  line L1632 (199.894, 47.7999) -> (199.1557, 48.5626)
  line L1633 (199.1683, 48.8371) -> (198.3134, 54.875)
  line L1634 (193.835, 54.875) -> (198.1134, 54.875)
  line L1635 (199.1557, 48.5626) -> (194.8169, 48.5626)
  line L1636 (198.3134, 54.875) -> (199.8283, 54.875)
  line L1637 (194.5288, 48.5624) -> (193.8558, 47.9125)
  line L1638 (7.7058, 72.5) -> (3.4274, 72.5)
  line L1639 (3.015, 74) -> (1.5, 74)
  arc A240 (10.6325, 59.875) -> (11.1276, 60.4451) centre (10.6325, 60.375) ccw
  circle A241 centre (1.5, 60.75) radius 0.875
  line L1640 (3.2642, 66.8375) -> (4.1602, 65.9119)
  line L1641 (9.7083, 59.875) -> (11.2083, 59.875)
  line L1642 (9.2939, 61.375) -> (5.0046, 61.375)
  line L1643 (4.1969, 67.6876) -> (3.4334, 66.9502)
  line L1644 (5.015, 59.875) -> (3.5, 59.875)
  line L1645 (3.5, 59.875) -> (2.5142, 66.8375)
  line L1646 (8.8126, 66.2013) -> (9.7083, 59.875)
  line L1647 (9.5063, 59.875) -> (9.2939, 61.375)
  line L1648 (8.5104, 66.1876) -> (9.274, 66.9249)
  line L1649 (10.1943, 67.0365) -> (9.4443, 67.0365)
  line L1650 (11.2083, 59.875) -> (10.2224, 66.8385)
  arc A242 (2.0758, 74) -> (1.5807, 73.4299) centre (2.0758, 73.5) ccw
  line L1651 (5.217, 59.875) -> (9.5063, 59.875)
  line L1652 (4.1602, 65.9119) -> (5.015, 59.875)
  line L1653 (9.4724, 66.8385) -> (8.8126, 66.2013)
  line L1654 (5.0046, 61.375) -> (5.217, 59.875)
  line L1655 (4.1717, 66.1876) -> (8.5104, 66.1876)
  line L1656 (9.4443, 67.0365) -> (8.5483, 67.9621)
  line L1657 (2.5142, 66.8375) -> (3.2642, 66.8375)
  line L1658 (10.2224, 66.8385) -> (9.4724, 66.8385)
  arc A243 (3.4391, 60.3049) -> (3.9342, 59.875) centre (3.9342, 60.375) ccw
  line L1659 (3.2358, 67.0375) -> (2.4858, 67.0375)
  line L1660 (7.4934, 74) -> (7.7058, 72.5)
  arc A244 (9.2692, 73.5701) -> (8.7741, 74) centre (8.7741, 73.5) ccw
  line L1661 (2.4858, 67.0375) -> (1.5, 74)
  line L1662 (3.4274, 72.5) -> (3.215, 74)
  line L1663 (9.2083, 74) -> (10.1943, 67.0365)
  line L1664 (3.4334, 66.9502) -> (4.1717, 66.1876)
  line L1665 (3.015, 74) -> (3.9088, 67.6874)
  line L1666 (9.274, 66.9249) -> (8.5357, 67.6876)
  line L1667 (8.5483, 67.9621) -> (7.6934, 74)
  line L1668 (3.215, 74) -> (7.4934, 74)
  line L1669 (8.5357, 67.6876) -> (4.1969, 67.6876)
  line L1670 (7.6934, 74) -> (9.2083, 74)
  line L1671 (3.9088, 67.6874) -> (3.2358, 67.0375)
  line L1672 (20.4138, 72.5) -> (16.1354, 72.5)
  line L1673 (15.723, 74) -> (14.208, 74)
  arc A245 (23.3405, 59.875) -> (23.8356, 60.4451) centre (23.3405, 60.375) ccw
  circle A246 centre (14.208, 60.75) radius 0.875
  line L1674 (15.9722, 66.8375) -> (16.8682, 65.9119)
  line L1675 (22.4163, 59.875) -> (23.9163, 59.875)
  line L1676 (22.0019, 61.375) -> (17.7126, 61.375)
  line L1677 (16.9049, 67.6876) -> (16.1414, 66.9502)
  line L1678 (17.723, 59.875) -> (16.208, 59.875)
  line L1679 (16.208, 59.875) -> (15.2222, 66.8375)
  line L1680 (21.5206, 66.2013) -> (22.4163, 59.875)
  line L1681 (22.2143, 59.875) -> (22.0019, 61.375)
  line L1682 (21.2184, 66.1876) -> (21.982, 66.9249)
  line L1683 (22.9023, 67.0365) -> (22.1523, 67.0365)
  line L1684 (23.9163, 59.875) -> (22.9304, 66.8385)
  arc A247 (14.7838, 74) -> (14.2887, 73.4299) centre (14.7838, 73.5) ccw
  line L1685 (17.925, 59.875) -> (22.2143, 59.875)
  line L1686 (16.8682, 65.9119) -> (17.723, 59.875)
  line L1687 (22.1804, 66.8385) -> (21.5206, 66.2013)
  line L1688 (17.7126, 61.375) -> (17.925, 59.875)
  line L1689 (16.8797, 66.1876) -> (21.2184, 66.1876)
  line L1690 (22.1523, 67.0365) -> (21.2563, 67.9621)
  line L1691 (15.2222, 66.8375) -> (15.9722, 66.8375)
  line L1692 (22.9304, 66.8385) -> (22.1804, 66.8385)
  arc A248 (16.1471, 60.3049) -> (16.6422, 59.875) centre (16.6422, 60.375) ccw
  line L1693 (15.9438, 67.0375) -> (15.1938, 67.0375)
  line L1694 (20.2014, 74) -> (20.4138, 72.5)
  arc A249 (21.9772, 73.5701) -> (21.4821, 74) centre (21.4821, 73.5) ccw
  line L1695 (15.1938, 67.0375) -> (14.208, 74)
  line L1696 (16.1354, 72.5) -> (15.923, 74)
  line L1697 (21.9163, 74) -> (22.9023, 67.0365)
  line L1698 (16.1414, 66.9502) -> (16.8797, 66.1876)
  line L1699 (15.723, 74) -> (16.6168, 67.6874)
  line L1700 (21.982, 66.9249) -> (21.2437, 67.6876)
  line L1701 (21.2563, 67.9621) -> (20.4014, 74)
  line L1702 (15.923, 74) -> (20.2014, 74)
  line L1703 (21.2437, 67.6876) -> (16.9049, 67.6876)
  line L1704 (20.4014, 74) -> (21.9163, 74)
  line L1705 (16.6168, 67.6874) -> (15.9438, 67.0375)
  line L1706 (33.1218, 72.5) -> (28.8434, 72.5)
  line L1707 (28.431, 74) -> (26.916, 74)
  arc A250 (36.0485, 59.875) -> (36.5436, 60.4451) centre (36.0485, 60.375) ccw
  circle A251 centre (26.916, 60.75) radius 0.875
  line L1708 (28.6802, 66.8375) -> (29.5762, 65.9119)
  line L1709 (35.1243, 59.875) -> (36.6243, 59.875)
  line L1710 (34.7099, 61.375) -> (30.4206, 61.375)
  line L1711 (29.6129, 67.6876) -> (28.8494, 66.9502)
  line L1712 (30.431, 59.875) -> (28.916, 59.875)
  line L1713 (28.916, 59.875) -> (27.9302, 66.8375)
  line L1714 (34.2286, 66.2013) -> (35.1243, 59.875)
  line L1715 (34.9223, 59.875) -> (34.7099, 61.375)
  line L1716 (33.9264, 66.1876) -> (34.69, 66.9249)
  line L1717 (35.6103, 67.0365) -> (34.8603, 67.0365)
  line L1718 (36.6243, 59.875) -> (35.6384, 66.8385)
  arc A252 (27.4918, 74) -> (26.9967, 73.4299) centre (27.4918, 73.5) ccw
  line L1719 (30.633, 59.875) -> (34.9223, 59.875)
  line L1720 (29.5762, 65.9119) -> (30.431, 59.875)
  line L1721 (34.8884, 66.8385) -> (34.2286, 66.2013)
  line L1722 (30.4206, 61.375) -> (30.633, 59.875)
  line L1723 (29.5877, 66.1876) -> (33.9264, 66.1876)
  line L1724 (34.8603, 67.0365) -> (33.9643, 67.9621)
  line L1725 (27.9302, 66.8375) -> (28.6802, 66.8375)
  line L1726 (35.6384, 66.8385) -> (34.8884, 66.8385)
  arc A253 (28.8551, 60.3049) -> (29.3502, 59.875) centre (29.3502, 60.375) ccw
  line L1727 (28.6518, 67.0375) -> (27.9018, 67.0375)
  line L1728 (32.9094, 74) -> (33.1218, 72.5)
  arc A254 (34.6852, 73.5701) -> (34.1901, 74) centre (34.1901, 73.5) ccw
  line L1729 (27.9018, 67.0375) -> (26.916, 74)
  line L1730 (28.8434, 72.5) -> (28.631, 74)
  line L1731 (34.6243, 74) -> (35.6103, 67.0365)
  line L1732 (28.8494, 66.9502) -> (29.5877, 66.1876)
  line L1733 (28.431, 74) -> (29.3248, 67.6874)
  line L1734 (34.69, 66.9249) -> (33.9517, 67.6876)
  line L1735 (33.9643, 67.9621) -> (33.1094, 74)
  line L1736 (28.631, 74) -> (32.9094, 74)
  line L1737 (33.9517, 67.6876) -> (29.6129, 67.6876)
  line L1738 (33.1094, 74) -> (34.6243, 74)
  line L1739 (29.3248, 67.6874) -> (28.6518, 67.0375)
  line L1740 (45.8298, 72.5) -> (41.5514, 72.5)
  line L1741 (41.139, 74) -> (39.624, 74)
  arc A255 (48.7565, 59.875) -> (49.2516, 60.4451) centre (48.7565, 60.375) ccw
  circle A256 centre (39.624, 60.75) radius 0.875
  line L1742 (41.3882, 66.8375) -> (42.2842, 65.9119)
  line L1743 (47.8323, 59.875) -> (49.3323, 59.875)
  line L1744 (47.4179, 61.375) -> (43.1286, 61.375)
  line L1745 (42.3209, 67.6876) -> (41.5574, 66.9502)
  line L1746 (43.139, 59.875) -> (41.624, 59.875)
  line L1747 (41.624, 59.875) -> (40.6382, 66.8375)
  line L1748 (46.9366, 66.2013) -> (47.8323, 59.875)
  line L1749 (47.6303, 59.875) -> (47.4179, 61.375)
  line L1750 (46.6344, 66.1876) -> (47.398, 66.9249)
  line L1751 (48.3183, 67.0365) -> (47.5683, 67.0365)
  line L1752 (49.3323, 59.875) -> (48.3464, 66.8385)
  arc A257 (40.1998, 74) -> (39.7047, 73.4299) centre (40.1998, 73.5) ccw
  line L1753 (43.341, 59.875) -> (47.6303, 59.875)
  line L1754 (42.2842, 65.9119) -> (43.139, 59.875)
  line L1755 (47.5964, 66.8385) -> (46.9366, 66.2013)
  line L1756 (43.1286, 61.375) -> (43.341, 59.875)
  line L1757 (42.2957, 66.1876) -> (46.6344, 66.1876)
  line L1758 (47.5683, 67.0365) -> (46.6723, 67.9621)
  line L1759 (40.6382, 66.8375) -> (41.3882, 66.8375)
  line L1760 (48.3464, 66.8385) -> (47.5964, 66.8385)
  arc A258 (41.5631, 60.3049) -> (42.0582, 59.875) centre (42.0582, 60.375) ccw
  line L1761 (41.3598, 67.0375) -> (40.6098, 67.0375)
  line L1762 (45.6174, 74) -> (45.8298, 72.5)
  arc A259 (47.3932, 73.5701) -> (46.8981, 74) centre (46.8981, 73.5) ccw
  line L1763 (40.6098, 67.0375) -> (39.624, 74)
  line L1764 (41.5514, 72.5) -> (41.339, 74)
  line L1765 (47.3323, 74) -> (48.3183, 67.0365)
  line L1766 (41.5574, 66.9502) -> (42.2957, 66.1876)
  line L1767 (41.139, 74) -> (42.0328, 67.6874)
  line L1768 (47.398, 66.9249) -> (46.6597, 67.6876)
  line L1769 (46.6723, 67.9621) -> (45.8174, 74)
  line L1770 (41.339, 74) -> (45.6174, 74)
  line L1771 (46.6597, 67.6876) -> (42.3209, 67.6876)
  line L1772 (45.8174, 74) -> (47.3323, 74)
  line L1773 (42.0328, 67.6874) -> (41.3598, 67.0375)
  line L1774 (58.5378, 72.5) -> (54.2594, 72.5)
  line L1775 (53.847, 74) -> (52.332, 74)
  arc A260 (61.4645, 59.875) -> (61.9596, 60.4451) centre (61.4645, 60.375) ccw
  circle A261 centre (52.332, 60.75) radius 0.875
  line L1776 (54.0962, 66.8375) -> (54.9922, 65.9119)
  line L1777 (60.5403, 59.875) -> (62.0403, 59.875)
  line L1778 (60.1259, 61.375) -> (55.8366, 61.375)
  line L1779 (55.0289, 67.6876) -> (54.2654, 66.9502)
  line L1780 (55.847, 59.875) -> (54.332, 59.875)
  line L1781 (54.332, 59.875) -> (53.3462, 66.8375)
  line L1782 (59.6446, 66.2013) -> (60.5403, 59.875)
  line L1783 (60.3383, 59.875) -> (60.1259, 61.375)
  line L1784 (59.3424, 66.1876) -> (60.106, 66.9249)
  line L1785 (61.0263, 67.0365) -> (60.2763, 67.0365)
  line L1786 (62.0403, 59.875) -> (61.0544, 66.8385)
  arc A262 (52.9078, 74) -> (52.4127, 73.4299) centre (52.9078, 73.5) ccw
  line L1787 (56.049, 59.875) -> (60.3383, 59.875)
  line L1788 (54.9922, 65.9119) -> (55.847, 59.875)
  line L1789 (60.3044, 66.8385) -> (59.6446, 66.2013)
  line L1790 (55.8366, 61.375) -> (56.049, 59.875)
  line L1791 (55.0037, 66.1876) -> (59.3424, 66.1876)
  line L1792 (60.2763, 67.0365) -> (59.3803, 67.9621)
  line L1793 (53.3462, 66.8375) -> (54.0962, 66.8375)
  line L1794 (61.0544, 66.8385) -> (60.3044, 66.8385)
  arc A263 (54.2711, 60.3049) -> (54.7662, 59.875) centre (54.7662, 60.375) ccw
  line L1795 (54.0678, 67.0375) -> (53.3178, 67.0375)
  line L1796 (58.3254, 74) -> (58.5378, 72.5)
  arc A264 (60.1012, 73.5701) -> (59.6061, 74) centre (59.6061, 73.5) ccw
  line L1797 (53.3178, 67.0375) -> (52.332, 74)
  line L1798 (54.2594, 72.5) -> (54.047, 74)
  line L1799 (60.0403, 74) -> (61.0263, 67.0365)
  line L1800 (54.2654, 66.9502) -> (55.0037, 66.1876)
  line L1801 (53.847, 74) -> (54.7408, 67.6874)
  line L1802 (60.106, 66.9249) -> (59.3677, 67.6876)
  line L1803 (59.3803, 67.9621) -> (58.5254, 74)
  line L1804 (54.047, 74) -> (58.3254, 74)
  line L1805 (59.3677, 67.6876) -> (55.0289, 67.6876)
  line L1806 (58.5254, 74) -> (60.0403, 74)
  line L1807 (54.7408, 67.6874) -> (54.0678, 67.0375)
  line L1808 (71.2458, 72.5) -> (66.9674, 72.5)
  line L1809 (66.555, 74) -> (65.04, 74)
  arc A265 (74.1725, 59.875) -> (74.6676, 60.4451) centre (74.1725, 60.375) ccw
  circle A266 centre (65.04, 60.75) radius 0.875
  line L1810 (66.8042, 66.8375) -> (67.7002, 65.9119)
  line L1811 (73.2483, 59.875) -> (74.7483, 59.875)
  line L1812 (72.8339, 61.375) -> (68.5446, 61.375)
  line L1813 (67.7369, 67.6876) -> (66.9734, 66.9502)
  line L1814 (68.555, 59.875) -> (67.04, 59.875)
  line L1815 (67.04, 59.875) -> (66.0542, 66.8375)
  line L1816 (72.3526, 66.2013) -> (73.2483, 59.875)
  line L1817 (73.0463, 59.875) -> (72.8339, 61.375)
  line L1818 (72.0504, 66.1876) -> (72.814, 66.9249)
  line L1819 (73.7343, 67.0365) -> (72.9843, 67.0365)
  line L1820 (74.7483, 59.875) -> (73.7624, 66.8385)
  arc A267 (65.6158, 74) -> (65.1207, 73.4299) centre (65.6158, 73.5) ccw
  line L1821 (68.757, 59.875) -> (73.0463, 59.875)
  line L1822 (67.7002, 65.9119) -> (68.555, 59.875)
  line L1823 (73.0124, 66.8385) -> (72.3526, 66.2013)
  line L1824 (68.5446, 61.375) -> (68.757, 59.875)
  line L1825 (67.7117, 66.1876) -> (72.0504, 66.1876)
  line L1826 (72.9843, 67.0365) -> (72.0883, 67.9621)
  line L1827 (66.0542, 66.8375) -> (66.8042, 66.8375)
  line L1828 (73.7624, 66.8385) -> (73.0124, 66.8385)
  arc A268 (66.9791, 60.3049) -> (67.4742, 59.875) centre (67.4742, 60.375) ccw
  line L1829 (66.7758, 67.0375) -> (66.0258, 67.0375)
  line L1830 (71.0334, 74) -> (71.2458, 72.5)
  arc A269 (72.8092, 73.5701) -> (72.3141, 74) centre (72.3141, 73.5) ccw
  line L1831 (66.0258, 67.0375) -> (65.04, 74)
  line L1832 (66.9674, 72.5) -> (66.755, 74)
  line L1833 (72.7483, 74) -> (73.7343, 67.0365)
  line L1834 (66.9734, 66.9502) -> (67.7117, 66.1876)
  line L1835 (66.555, 74) -> (67.4488, 67.6874)
  line L1836 (72.814, 66.9249) -> (72.0757, 67.6876)
  line L1837 (72.0883, 67.9621) -> (71.2334, 74)
  line L1838 (66.755, 74) -> (71.0334, 74)
  line L1839 (72.0757, 67.6876) -> (67.7369, 67.6876)
  line L1840 (71.2334, 74) -> (72.7483, 74)
  line L1841 (67.4488, 67.6874) -> (66.7758, 67.0375)
  line L1842 (83.9538, 72.5) -> (79.6754, 72.5)
  line L1843 (79.263, 74) -> (77.748, 74)
  arc A270 (86.8805, 59.875) -> (87.3756, 60.4451) centre (86.8805, 60.375) ccw
  circle A271 centre (77.748, 60.75) radius 0.875
  line L1844 (79.5122, 66.8375) -> (80.4082, 65.9119)
  line L1845 (85.9563, 59.875) -> (87.4563, 59.875)
  line L1846 (85.5419, 61.375) -> (81.2526, 61.375)
  line L1847 (80.4449, 67.6876) -> (79.6814, 66.9502)
  line L1848 (81.263, 59.875) -> (79.748, 59.875)
  line L1849 (79.748, 59.875) -> (78.7622, 66.8375)
  line L1850 (85.0606, 66.2013) -> (85.9563, 59.875)
  line L1851 (85.7543, 59.875) -> (85.5419, 61.375)
  line L1852 (84.7584, 66.1876) -> (85.522, 66.9249)
  line L1853 (86.4423, 67.0365) -> (85.6923, 67.0365)
  line L1854 (87.4563, 59.875) -> (86.4704, 66.8385)
  arc A272 (78.3238, 74) -> (77.8287, 73.4299) centre (78.3238, 73.5) ccw
  line L1855 (81.465, 59.875) -> (85.7543, 59.875)
  line L1856 (80.4082, 65.9119) -> (81.263, 59.875)
  line L1857 (85.7204, 66.8385) -> (85.0606, 66.2013)
  line L1858 (81.2526, 61.375) -> (81.465, 59.875)
  line L1859 (80.4197, 66.1876) -> (84.7584, 66.1876)
  line L1860 (85.6923, 67.0365) -> (84.7963, 67.9621)
  line L1861 (78.7622, 66.8375) -> (79.5122, 66.8375)
  line L1862 (86.4704, 66.8385) -> (85.7204, 66.8385)
  arc A273 (79.6871, 60.3049) -> (80.1822, 59.875) centre (80.1822, 60.375) ccw
  line L1863 (79.4838, 67.0375) -> (78.7338, 67.0375)
  line L1864 (83.7414, 74) -> (83.9538, 72.5)
  arc A274 (85.5172, 73.5701) -> (85.0221, 74) centre (85.0221, 73.5) ccw
  line L1865 (78.7338, 67.0375) -> (77.748, 74)
  line L1866 (79.6754, 72.5) -> (79.463, 74)
  line L1867 (85.4563, 74) -> (86.4423, 67.0365)
  line L1868 (79.6814, 66.9502) -> (80.4197, 66.1876)
  line L1869 (79.263, 74) -> (80.1568, 67.6874)
  line L1870 (85.522, 66.9249) -> (84.7837, 67.6876)
  line L1871 (84.7963, 67.9621) -> (83.9414, 74)
  line L1872 (79.463, 74) -> (83.7414, 74)
  line L1873 (84.7837, 67.6876) -> (80.4449, 67.6876)
  line L1874 (83.9414, 74) -> (85.4563, 74)
  line L1875 (80.1568, 67.6874) -> (79.4838, 67.0375)
  line L1876 (96.6618, 72.5) -> (92.3834, 72.5)
  line L1877 (91.971, 74) -> (90.456, 74)
  arc A275 (99.5885, 59.875) -> (100.0836, 60.4451) centre (99.5885, 60.375) ccw
  circle A276 centre (90.456, 60.75) radius 0.875
  line L1878 (92.2202, 66.8375) -> (93.1162, 65.9119)
  line L1879 (98.6643, 59.875) -> (100.1643, 59.875)
  line L1880 (98.2499, 61.375) -> (93.9606, 61.375)
  line L1881 (93.1529, 67.6876) -> (92.3894, 66.9502)
  line L1882 (93.971, 59.875) -> (92.456, 59.875)
  line L1883 (92.456, 59.875) -> (91.4702, 66.8375)
  line L1884 (97.7686, 66.2013) -> (98.6643, 59.875)
  line L1885 (98.4623, 59.875) -> (98.2499, 61.375)
  line L1886 (97.4664, 66.1876) -> (98.23, 66.9249)
  line L1887 (99.1503, 67.0365) -> (98.4003, 67.0365)
  line L1888 (100.1643, 59.875) -> (99.1784, 66.8385)
  arc A277 (91.0318, 74) -> (90.5367, 73.4299) centre (91.0318, 73.5) ccw